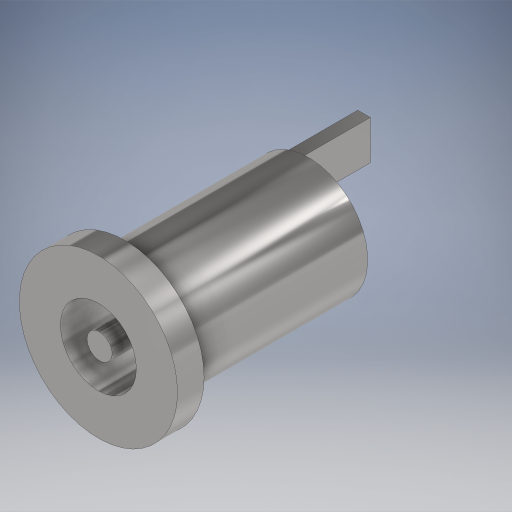
# Autodesk Inventor part: Разъём питания
Saved by Autodesk Inventor 2023 (Build 270158000, 158)
## iProperties
Created: 2023-01-04
Part Number: Разъём питания
Material: Типовые
Document SubType Name: Modeling
Designer: Admin
Density: 1 g/cm^3
Appearance: По умолчанию
Author: Admin
Autodesk Inventor part; units mm, degrees
ref_plane "YZ Plane" through (0, 0, 0) normal (1, 0, 0) x (0, 1, 0)
ref_plane "XZ Plane" through (0, 0, 0) normal (0, 1, 0) x (-1, 0, 0)
ref_plane "XY Plane" through (0, 0, 0) normal (0, 0, 1) x (1, 0, 0)
sketch "Эскиз1" plane through (0, 0, 0) normal (0, 0, 1) x (1, 0, 0)
  circle A0 centre (0, 0) radius 6.25
  circle A1 centre (0, 0) radius 4.675
  circle A2 centre (0, 0) radius 1
  circle A3 centre (0, 0) radius 3
  dimension "d0" = 12.5
  dimension "d1" = 9.35
  dimension "d2" = 6
  dimension "d3" = 2
  constraints: 4 centre point, 4 coincident
  measures "d0" diameter of A0
  measures "d1" diameter of A1
  measures "d2" diameter of A3
  measures "d3" diameter of A2
extrude "Выдавливание1" add sketch "Эскиз1" along normal blind 2.1 contours A0 | A1 | A2 | A3
extrude "Выдавливание2" add sketch "Эскиз1" against normal blind 14.5 contours A1 | A2 | A3
sketch "Эскиз2" plane through (0, 0, -14.5) normal (0, 0, -1) x (-1, 0, 0)
  circle A0 centre (0, 0) radius 6.25
  line L0 (4.41057, 1.55) -> (4.41057, -1.55)
  line L1 (3.41057, 1.55) -> (3.41057, -1.55)
  line L2 (3.41057, 1.55) -> (4.41057, 1.55)
  line L3 (3.41057, -1.55) -> (4.41057, -1.55)
  circle A1 centre (0, 0) radius 4.675
  dimension "d8" = 3.1
  dimension "d9" = 1
  constraints: 8 end point, 2 parallel, 2 point on circle, 2 vertical, 1 horizontal
  measures "d8" distance of L1.start L1.end
  measures "d9" distance between parallel lines of L0 L1
extrude "Выдавливание3" add sketch "Эскиз2" along normal blind 8.3 contours L0 L3 L1 L2
extrude "Выдавливание4" cut sketch "Эскиз1" along normal mid plane 5 contours A2 | A3
extrude "Выдавливание5" add sketch "Эскиз1" along normal blind 2 and the other way blind 5 contours A2
fillet "Сопряжение1" radius 1 1 edges at (-4.4106, 0, -14.5)
